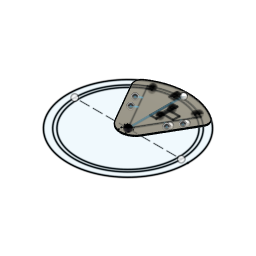
funnel_panel v7 (Autodesk Fusion 360 design; units mm, degrees)
Autodesk Fusion 360 part; units mm, degrees
sketch "Sketch1" plane through (0, 0, 0) normal (0, 0, 1) x (1, 0, 0)
  line L0 (35, 260) -> (35, 180)
  circle A0 centre (35, 260) radius 2.5
  circle A1 centre (35, 180) radius 2.5
  line L1 (0, 290) -> (40, 290)
  line L2 (40, 290) -> (40, 150)
  line L3 (40, 150) -> (0, 150)
  line L4 (0, 150) -> (0, 290)
  line L5 (25, 241) -> (103, 241)
  line L6 (103, 241) -> (103, 199)
  line L7 (103, 199) -> (25, 199)
  line L8 (25, 199) -> (25, 241)
  line L9 (0, 0) -> (0, 372.5)
  circle A2 centre (35, 180) radius 2.5
  line L10 (0, 0) -> (0, 372.5)
  line L11 (40, 150) -> (0, 150)
  line L12 (25, 241) -> (103, 241)
  line L13 (0, 150) -> (0, 290)
  line L14 (40, 290) -> (40, 150)
  line L15 (103, 241) -> (103, 199)
  line L16 (103, 199) -> (25, 199)
  line L17 (0, 290) -> (40, 290)
  line L18 (25, 199) -> (25, 241)
  circle A3 centre (35, 260) radius 2.5
  line L19 (35, 260) -> (35, 180)
  circle A4 centre (0, 0) radius 356.25
  circle A5 centre (0, 0) radius 336.25
  line L20 (0, 0) -> (178.125, 308.5216)
  line L21 (0, 0) -> (356.25, 0) construction
  line L22 (130, 225.1666) -> (160.3109, 207.6666)
  line L23 (130, 225.1666) -> (165, 225.1666) construction
  line L24 (90, 155.8846) -> (120.3109, 138.3846)
  line L25 (90, 155.8846) -> (125, 155.8846) construction
  circle A6 centre (160.3109, 207.6666) radius 2.5
  circle A7 centre (120.3109, 138.3846) radius 2.5
  line L26 (0, 0) -> (-178.125, 308.5216)
  line L27 (0, 0) -> (-356.25, 0) construction
  line L28 (-130, 225.1666) -> (-160.3109, 207.6666)
  line L29 (-90, 155.8846) -> (-120.3109, 138.3846)
  circle A8 centre (-160.3109, 207.6666) radius 2.5
  circle A9 centre (-120.3109, 138.3846) radius 2.5
  circle A10 centre (0, 0) radius 400
  line L30 (-44, 372.5) -> (-10, 372.5)
  line L31 (-10, 372.5) -> (-10, 320)
  line L32 (-10, 320) -> (-44, 320)
  line L33 (-44, 320) -> (-44, 372.5)
  line L34 (0, 356.25) -> (-27, 356.25)
  line L35 (0, 336.25) -> (-27, 336.25)
  circle A11 centre (-27, 356.25) radius 1.6
  circle A12 centre (-27, 336.25) radius 1.6
  line L36 (-178.125, 308.5216) -> (-154.7423, 322.0216)
  line L37 (-168.125, 291.201) -> (-144.7423, 304.701)
  circle A13 centre (-154.7423, 322.0216) radius 1.6
  circle A14 centre (-144.7423, 304.701) radius 1.6
  line L38 (178.125, 308.5216) -> (154.7423, 322.0216)
  line L39 (168.125, 291.201) -> (144.7423, 304.701)
  circle A15 centre (144.7423, 304.701) radius 1.6
  circle A16 centre (154.7423, 322.0216) radius 1.6
  dimension "d13" = 80
  dimension "d14" = 5
  dimension "d15" = 5
  dimension "d16" = 35
  dimension "d17" = 40
  dimension "d18" = 140
  dimension "d19" = 35
  dimension "d22" = 150
  dimension "d23" = 30
  dimension "d25" = 78
  dimension "d26" = 42
  dimension "d27" = 25
  dimension "d28" = 49
  dimension "d36" = 80
  dimension "d37" = 5
  dimension "d38" = 5
  dimension "d39" = 35
  dimension "d40" = 40
  dimension "d41" = 140
  dimension "d42" = 35
  dimension "d44" = 150
  dimension "d45" = 30
  dimension "d47" = 78
  dimension "d48" = 42
  dimension "d49" = 25
  dimension "d50" = 49
  dimension "d51" = 60
  dimension "d54" = 30
  dimension "d55" = 35
  dimension "d56" = 30
  dimension "d57" = 35
  dimension "d59" = 80
  dimension "d60" = 5
  dimension "d61" = 5
  dimension "d62" = 60
  dimension "d65" = 35
  dimension "d66" = 35
  dimension "d68" = 80
  dimension "d69" = 5
  dimension "d70" = 5
  dimension "d123" = 34
  dimension "d124" = 52.5
  dimension "d126" = 10
  dimension "d127" = 30
  dimension "d128" = 27
  dimension "d129" = 27
  dimension "d130" = 3.2
  dimension "d131" = 3.2
  dimension "d132" = 712.5
  dimension "d133" = 672.5
  dimension "d134" = 800
  dimension "d137" = 3.2
  dimension "d138" = 3.2
  dimension "d139" = 27
  dimension "d140" = 27
  dimension "d141" = 3.2
  dimension "d142" = 3.2
  dimension "d143" = 27
  dimension "d144" = 27
  constraint vertical L0
  constraint coincident L0.start A0.centre
  constraint coincident L0.end A1.centre
  constraint horizontal L1
  constraint vertical L2
  constraint horizontal L3
  constraint vertical L4
  constraint horizontal L5
  constraint vertical L6
  constraint horizontal L7
  constraint vertical L8
  constraint coincident L9.start L10.start
  constraint vertical L19
  constraint horizontal L17
  constraint vertical L14
  constraint horizontal L11
  constraint vertical L13
  constraint horizontal L12
  constraint vertical L15
  constraint horizontal L16
  constraint vertical L18
  constraint horizontal L21
  constraint coincident A4 L20.end
  constraint horizontal L23
  constraint coincident L20 L22.start
  constraint horizontal L25
  constraint coincident L20 L24.start
  constraint coincident L22.end A6.centre
  constraint coincident L24.end A7.centre
  constraint horizontal L27
  constraint coincident A4 L26.end
  constraint coincident L26 L28.start
  constraint perpendicular L26 L28
  constraint coincident L26 L29.start
  constraint perpendicular L26 L29
  constraint coincident L28.end A8.centre
  constraint coincident L29.end A9.centre
  constraint horizontal L30
  constraint vertical L31
  constraint horizontal L32
  constraint vertical L33
  constraint coincident L10 L34.start
  constraint coincident A4 L34.start
  constraint perpendicular L31 L34
  constraint coincident L10 L35.start
  constraint coincident A5 L35.start
  constraint perpendicular L31 L35
  constraint coincident L34.end A11.centre
  constraint coincident L35.end A12.centre
  constraint perpendicular L26 L36
  constraint coincident A5 L37.start
  constraint coincident L26 L37.start
  constraint perpendicular L26 L37
  constraint coincident L36.end A13.centre
  constraint coincident L37.end A14.centre
  constraint perpendicular L20 L38
  constraint coincident A5 L39.start
  constraint coincident L20 L39.start
  constraint tangent A5 L39
  constraint perpendicular L20 L39
  constraint coincident L39.end A15.centre
  constraint coincident L38.end A16.centre
  constraint concentric A4 A5
  measures "d13" distance of L0.start L0.end
  measures "d14" diameter of A0
  measures "d15" diameter of A1
  measures "d16" distance of L9.start L0
  measures "d17" distance of L1.start L1.end
  measures "d18" distance of L1.start L3.end
  measures "d19" distance of L0.start L4
  measures "d22" distance of L9.start L3
  measures "d23" distance of L0.start L1
  measures "d25" distance of L5.start L5.end
  measures "d26" distance of L5.start L7.end
  measures "d27" distance of L4 L8
  measures "d28" distance of L3 L7
  measures "d36" distance of L0.end L0.start
  measures "d37" diameter of A3
  measures "d38" diameter of A2
  measures "d39" distance of L9.start L19
  measures "d40" distance of L1.end L1.start
  measures "d41" distance of L3.end L1.start
  measures "d42" distance of L0.start L13
  measures "d44" distance of L9.start L11
  measures "d45" distance of L0.start L17
  measures "d47" distance of L5.start L5.end
  measures "d48" distance of L5.start L7.end
  measures "d49" distance of L13 L18
  measures "d50" distance of L11 L16
  measures "d51" angle of L20 L21
  measures "d54" angle of L22 L23
  measures "d55" distance of L22.start L22.end
  measures "d56" angle of L24 L25
  measures "d57" distance of L24.start L24.end
  measures "d59" distance of L22 L24
  measures "d60" diameter of A6
  measures "d61" diameter of A7
  measures "d62" angle of L26 L27
  measures "d65" distance of L28.start L28.end
  measures "d66" distance of L29.start L29.end
  measures "d68" distance of L28 L29
  measures "d69" diameter of A8
  measures "d70" diameter of A9
  measures "d123" distance of L30.start L30.end
  measures "d124" distance of L30.start L32.end
  measures "d126" distance of L10 L31
  measures "d127" distance of L1 L32
  measures "d128" distance of L34.start L34.end
  measures "d129" distance of L35.start L35.end
  measures "d130" diameter of A11
  measures "d131" diameter of A12
  measures "d132" diameter of A4
  measures "d133" diameter of A5
  measures "d134" diameter of A10
  measures "d137" diameter of A13
  measures "d138" diameter of A14
  measures "d139" distance of L20.end L38.end
  measures "d140" distance of L39.start L39.end
  measures "d141" diameter of A15
  measures "d142" diameter of A16
  measures "d143" distance of L37.start L37.end
  measures "d144" distance of L26.end L36.end
extrude "Extrude1" add sketch "Sketch1" along normal blind 5 contours L0 L2 L5 L7 L12 L14 L16 L19 | L0 L5 L7 L8 L12 L16 L18 L19 | L1 L2 L3 L4 L5 L7 L8 L9 L10 L11 L12 L13 L14 L16 L17 L18 | L2 L5 L6 L7 L12 L14 L15 L16 | L1 L2 L3 L5 L6 L7 L9 L10 L11 L12 L14 L15 L16 L17 A5 L20 A15 | L4 L9 L10 L13 A5 L26 L31 L32 L33 A14 | L9 L10 A4 L31 L35 | L9 L10 A4 A5 L20 L39 A15 A16 | A5 L31 L35 | A5 L20 L26 | A4 L31 L34 | A5 L31 L32 L33 A12 | A5 L31 L35 A12 | A4 A5 L31 L33 L35 A11 A12 | A4 L31 L34 A11 | A4 L30 L31 L33 L34 A11 | A5 L39 A15 | A4 L38 A16 | A4 A5 L20 L26 | A5 L37 A14 | A4 A5 L26 L33 L37 A13 A14 | A4 L36 A13 | A10
sketch "Sketch2" plane through (0, 0, 5) normal (0, 0, 1) x (-1, 0, 0)
  circle A0 centre (-160.3109, -207.6666) radius 2.5
  circle A1 centre (160.3109, -207.6666) radius 2.5
  circle A2 centre (120.3109, -138.3846) radius 2.5
  circle A3 centre (-35, -180) radius 2.5
  circle A4 centre (-120.3109, -138.3846) radius 2.5
  circle A5 centre (-35, -260) radius 2.5
  circle A6 centre (0, 0) radius 400
  line L0 (-86.6025, 0) -> (-261.4048, -302.7664)
  line L1 (-86.6025, 0) -> (197.573, 0) construction
  line L2 (86.6025, 0) -> (261.4048, -302.7664)
  line L3 (86.6025, 0) -> (440.5125, 0) construction
  line L4 (0, -400) -> (0, 0)
  line L5 (0, 0) -> (200, -346.4102)
  line L6 (0, 0) -> (400, 0) construction
  line L7 (0, 0) -> (-200, -346.4102)
  arc A7 (86.6025, 0) -> (-86.6025, 0) centre (0, -50) ccw
  circle A8 centre (-144.7423, -304.701) radius 1.6
  circle A9 centre (-154.7423, -322.0216) radius 1.6
  circle A10 centre (154.7423, -322.0216) radius 1.6
  circle A11 centre (27, -336.25) radius 1.6
  circle A12 centre (27, -356.25) radius 1.6
  circle A13 centre (144.7423, -304.701) radius 1.6
  dimension "d73" = 120
  dimension "d74" = 40
  dimension "d75" = 60
  dimension "d76" = 40
  dimension "d77" = 60
  dimension "d78" = 120
  constraint horizontal L1
  constraint coincident A6 L0.end
  constraint horizontal L3
  constraint coincident L1 L2.start
  constraint coincident A6 L2.end
  constraint coincident A6 L4.start
  constraint coincident A6.centre L4.end
  constraint perpendicular L1 L4
  constraint horizontal L6
  constraint coincident A6 L5.end
  constraint coincident A6 L7.end
  measures "d73" angle of L0 L1
  measures "d74" distance of A0.centre L0
  measures "d75" angle of L2 L3
  measures "d76" distance of A1.centre L2
  measures "d77" angle of L5 L6
  measures "d78" angle of L5 L7
extrude "Extrude2" cut sketch "Sketch2" against normal blind 5 contours A6 L0 L2 A7
sketch "Sketch3" plane through (0, 0, 5) normal (0, 0, 1) x (-1, 0, 0)
  line L0 (-86.6025, 0) -> (-261.4048, -302.7664)
  arc A0 (-261.4048, -302.7664) -> (261.4048, -302.7664) centre (0, 0) ccw
  line L1 (261.4048, -302.7664) -> (86.6025, 0)
  arc A1 (86.6025, 0) -> (-86.6025, 0) centre (0, -50) ccw
  circle A2 centre (-160.3109, -207.6666) radius 2.5
  circle A3 centre (160.3109, -207.6666) radius 2.5
  circle A4 centre (120.3109, -138.3846) radius 2.5
  circle A5 centre (-35, -180) radius 2.5
  circle A6 centre (-120.3109, -138.3846) radius 2.5
  circle A7 centre (-35, -260) radius 2.5
  line L2 (0, 0) -> (0, -400)
  line L3 (0, 0) -> (-200, -346.4102)
  line L4 (0, 0) -> (200, -346.4102)
  line L5 (0, 0) -> (400, 0) construction
  circle A8 centre (15, -5.9808) radius 10
  circle A9 centre (-15, -5.9808) radius 10
  line L6 (0, 0) -> (0, 50)
  line L7 (5, -5.9808) -> (5, 49.8749)
  line L8 (-5, -5.9808) -> (-5, 49.8749)
  line L9 (-15, -5.9808) -> (-22.5, -18.9711)
  line L10 (-15, -5.9808) -> (0, -5.9808) construction
  line L11 (-15, -5.9808) -> (-30, -5.9808)
  circle A10 centre (-22.5, -18.9711) radius 1.6
  circle A11 centre (-30, -5.9808) radius 1.6
  line L12 (15, -5.9808) -> (22.5, -18.9711)
  line L13 (15, -5.9808) -> (30, -5.9808) construction
  line L14 (15, -5.9808) -> (30, -5.9808)
  circle A12 centre (22.5, -18.9711) radius 1.6
  circle A13 centre (30, -5.9808) radius 1.6
  circle A14 centre (-144.7423, -304.701) radius 1.6
  circle A15 centre (-154.7423, -322.0216) radius 1.6
  circle A16 centre (154.7423, -322.0216) radius 1.6
  circle A17 centre (27, -336.25) radius 1.6
  circle A18 centre (27, -356.25) radius 1.6
  circle A19 centre (144.7423, -304.701) radius 1.6
  dimension "d81" = 150
  dimension "d82" = 60
  dimension "d83" = 20
  dimension "d84" = 20
  dimension "d87" = 5
  dimension "d88" = 5
  dimension "d89" = 120
  dimension "d90" = 15
  dimension "d91" = 15
  dimension "d92" = 3.2
  dimension "d93" = 3.2
  dimension "d94" = 60
  dimension "d95" = 15
  dimension "d96" = 3.2
  dimension "d97" = 3.2
  constraint coincident A0.centre L2.start
  constraint midpoint A0 L2.end
  constraint coincident A0 L3.end
  constraint horizontal L5
  constraint coincident A0 L4.end
  constraint tangent L4 A8
  constraint tangent L3 A9
  constraint midpoint A1 L6.end
  constraint coincident A8 L7.start
  constraint coincident A1 L7.end
  constraint tangent A8 L7
  constraint parallel L6 L7
  constraint coincident A9 L8.start
  constraint coincident A1 L8.end
  constraint tangent A9 L8
  constraint vertical L8
  constraint horizontal L10
  constraint coincident A9.centre L9.start
  constraint parallel L10 L11
  constraint coincident L9.end A10.centre
  constraint coincident L11.end A11.centre
  constraint horizontal L13
  constraint coincident A8.centre L12.start
  constraint parallel L13 L14
  constraint coincident L12.end A12.centre
  constraint coincident L13.end L14.end
  measures "d81" angle of L2 L3
  measures "d82" angle of L4 L5
  measures "d83" diameter of A8
  measures "d84" diameter of A9
  measures "d87" distance of L6 L7
  measures "d88" distance of L6 L8
  measures "d89" angle of L9 L10
  measures "d90" distance of A9.centre L9.end
  measures "d91" distance of A9.centre L11.end
  measures "d92" diameter of A10
  measures "d93" diameter of A11
  measures "d94" angle of L12 L13
  measures "d95" distance of A8.centre L12.end
  measures "d96" diameter of A12
  measures "d97" diameter of A13
extrude "Extrude3" cut sketch "Sketch3" against normal blind 5 contours A10 | A11 | A12 | A13
sketch "Sketch4" plane through (0, 0, 5) normal (0, 0, 1) x (-1, 0, 0)
  circle A0 centre (30, -5.9808) radius 1.6
  circle A1 centre (-22.5, -18.9711) radius 1.6
  circle A2 centre (22.5, -18.9711) radius 1.6
  circle A3 centre (-30, -5.9808) radius 1.6
  line L0 (-86.6025, 0) -> (-261.4048, -302.7664)
  arc A4 (-261.4048, -302.7664) -> (261.4048, -302.7664) centre (0, 0) ccw
  line L1 (261.4048, -302.7664) -> (86.6025, 0)
  arc A5 (86.6025, 0) -> (-86.6025, 0) centre (0, -50) ccw
  circle A6 centre (-160.3109, -207.6666) radius 2.5
  circle A7 centre (160.3109, -207.6666) radius 2.5
  circle A8 centre (120.3109, -138.3846) radius 2.5
  circle A9 centre (-35, -180) radius 2.5
  circle A10 centre (-120.3109, -138.3846) radius 2.5
  circle A11 centre (-35, -260) radius 2.5
  line L2 (0, 50) -> (0, -25)
  line L3 (-5, -25) -> (-5, 49.8749)
  line L4 (5, -25) -> (5, 49.8749)
  line L5 (23, 20) -> (-23, 20)
  line L6 (-23, 20) -> (-23, 40)
  line L7 (-23, 40) -> (23, 40)
  line L8 (23, 40) -> (23, 20)
  circle A12 centre (21.4, 20) radius 1.6
  circle A13 centre (24.6, 20) radius 1.6
  line L9 (21.4, 21.6) -> (24.6, 21.6)
  line L10 (24.6, 18.4) -> (21.4, 18.4)
  circle A14 centre (-21.4, 20) radius 1.6
  circle A15 centre (-24.6, 20) radius 1.6
  line L11 (-21.4, 18.4) -> (-24.6, 18.4)
  line L12 (-24.6, 21.6) -> (-21.4, 21.6)
  circle A16 centre (24.6, 40) radius 1.6
  circle A17 centre (21.4, 40) radius 1.6
  line L13 (24.6, 38.4) -> (21.4, 38.4)
  line L14 (21.4, 41.6) -> (24.6, 41.6)
  circle A18 centre (-21.4, 40) radius 1.6
  circle A19 centre (-24.6, 40) radius 1.6
  line L15 (-21.4, 38.4) -> (-24.6, 38.4)
  line L16 (-24.6, 41.6) -> (-21.4, 41.6)
  circle A20 centre (-144.7423, -304.701) radius 1.6
  circle A21 centre (-154.7423, -322.0216) radius 1.6
  circle A22 centre (154.7423, -322.0216) radius 1.6
  circle A23 centre (27, -336.25) radius 1.6
  circle A24 centre (27, -356.25) radius 1.6
  circle A25 centre (144.7423, -304.701) radius 1.6
  dimension "d100" = 5
  dimension "d101" = 5
  dimension "d102" = 46
  dimension "d103" = 20
  dimension "d104" = 10
  dimension "d105" = 23
  dimension "d107" = 3.2
  dimension "d108" = 3.2
  dimension "d111" = -46
  dimension "d112" = 20
  constraint midpoint A5 L2.start
  constraint vertical L2
  constraint coincident A5 L3.end
  constraint vertical L3
  constraint coincident A5 L4.end
  constraint parallel L2 L4
  constraint horizontal L5
  constraint vertical L6
  constraint horizontal L7
  constraint vertical L8
  constraint coincident L5 A12.centre
  constraint tangent L8 A12
  constraint tangent L8 A13
  constraint coincident A12 L9.start
  constraint coincident A13 L9.end
  constraint tangent A13 L9
  constraint coincident A13 L10.start
  constraint coincident A12 L10.end
  constraint tangent A12 L10
  constraint parallel L9 L10
  measures "d100" distance of L2 L4
  measures "d101" distance of L2 L3
  measures "d102" distance of L5.start L5.end
  measures "d103" distance of L5.start L7.end
  measures "d104" distance of L2.start L7
  measures "d105" distance of L2 L6
  measures "d107" diameter of A12
  measures "d108" diameter of A13
extrude "Extrude4" cut sketch "Sketch4" against normal blind 5 contours L7 A18 | L7 A18 | L5 A14 | L5 A14 | L6 A18 L15 | A18 A19 L16 | A19 | L6 A19 L15 | L7 A17 | L7 A17 | L6 A15 L12 | L6 A14 L12 | A15 | A14 A15 L11 | L5 A12 | L5 A12 | L8 A16 L13 | A16 A17 L14 | A16 | L8 A17 L13 | L8 A12 L9 | A12 A13 L10 | L8 A13 L9 | A13
fillet "Fillet1" radius 50 2 edges at (261.4048, 302.7664, 2.5) (-261.4048, 302.7664, 2.5)
